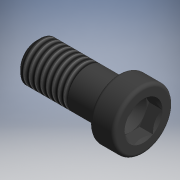
# Autodesk Inventor part: DIN-6912 - M12x25(F)
Saved by Autodesk Inventor 2017.3 (Build 213256000, 256)
## iProperties
Part Number: DIN-6912 - M12x25(F)
Material: Generic
Catalog Web Link: www.cadenas.de
Description: DIN-6912-Hexagon socket head cap screw with centre hole and low head
Vendor: FESTO
Document SubType Name: Modeling
Designer: partserver
Manufacturer: FESTO
Mass: 4.1242 g
Surface Area: 20.1844 cm^2
Volume: 4.1242 cm^3
Density: 1 g/cm^3
Appearance: PSOLRGB-80-80-80
Category: PARTsolutions
Company: FESTO
Title: DIN-6912 - M12x25(F)
Author: Cadenas PARTsolutions
Comments: Hexagon socket head cap screw with centre hole and low head
PSOL_IDENT_0: {$CADENAS_DATA\23d-libs\festo\zyl_zubeh\din_6912\din_6912.prj},183 {VTYP=3D},{NB=DIN-6912 - M12x25(F
PSOL_IDENT_1: )},{LINA=DIN-6912 - M12x25(F)},{NN=DIN-6912},{DATE=16.11.2017 11:29:57},{GEOMDATE=16.11.2017 11:29:4
PSOL_IDENT_2: 4},{VERSION=},{LINEID=550},{WBVAR=},{WBNUMERIC=}  {NB=DIN-6912 - M12x25(F)},{LINA=DIN-6912 - M12x25(
PSOL_IDENT_3: F)},{KT=L},{IDNR=},{NENN=M12x25},{D=12.000},{L=25.000},{DK=9.853},{LS=4.200},{LG=9.500},{DK1=18.000}
PSOL_IDENT_4: ,{DH=6.000},{K=7.500},{R=0.600},{V=1.000},{S=10.000},{T1=4.000},{T2=9.000},{F=1.450},{DA=13.700},{DW=
PSOL_IDENT_5: 17.030}
NB: DIN-6912 - M12x25(F)
NN: DIN-6912
NT: Hexagon socket head cap screw with centre hole and low head
NBSYN: DIN-6912 - $NENN.(F)
LINA: DIN-6912 - M12x25(F)
CATALOG: Festo
ROWDESC: M12x25
D: 12
L: 25
DK: 9.853
LS: 4.2
LG: 9.5
DK1: 18
DH: 6
K: 7.5
R: 0.6
V: 1
S: 10
T1: 4
T2: 9
F: 1.45
DA: 13.7
DW: 17.03
SUPPLIER: FESTO
ARTICLENO: DIN-6912 - M12x25(F)
BOMINFO: DIN-6912 - M12x25(F)
CREATOR: CADENAS GmbH
Autodesk Inventor part; units mm, degrees
sketch "Sketch_1" plane through (0, 0, 0) normal (0, 0, 1) x (1, 0, 0)
  line L0 (25, 0) -> (4.5, 0)
  line L1 (4.5, 0) -> (1.5, 3)
  line L2 (1.5, 3) -> (-1.5, 3)
  line L3 (-1.5, 3) -> (-3.5, 5)
  line L4 (-3.5, 5) -> (-6.7265, 5)
  line L5 (-6.7265, 5) -> (-7.5, 5.7735)
  line L6 (-7.5, 5.7735) -> (-7.5, 8)
  arc A0 (-6.5, 9) -> (-7.5, 8) centre (-6.5, 8) ccw
  line L7 (-6.5, 9) -> (-1, 9)
  arc A1 (0, 8) -> (-1, 9) centre (-1, 8) ccw
  line L8 (0, 8) -> (0, 6)
  line L9 (0, 6) -> (23.9265, 6)
  line L10 (23.9265, 6) -> (25, 4.9265)
  line L11 (25, 4.9265) -> (25, 0)
  line L12 (25, 0) -> (4.5, 0)
  constraints: 26 end point, 4 point on circle, 2 centre point
revolve "Revolution1" add sketch "Sketch_1" angle 360 about axis through (25, 0, 0) along (-1, 0, 0)
thread "Thread1" size "M12x1.75" class "6g" standard "ISO Metric profile" length 14.4265
sketch "Sketch_2" plane through (-7.5, 0, 0) normal (1, 0, 0) x (0, 0, -1)
  line L0 (-5, -2.8868) -> (0, -5.7735)
  line L1 (0, -5.7735) -> (5, -2.8868)
  line L2 (5, -2.8868) -> (5, 2.8868)
  line L3 (5, 2.8868) -> (0, 5.7735)
  line L4 (0, 5.7735) -> (-5, 2.8868)
  line L5 (-5, 2.8868) -> (-5, -2.8868)
  constraints: 12 end point
extrude "Extrusion1" cut sketch "Sketch_2" along normal blind 4
ref_plane "MONTAGE_XY" through (0, 0, 0) normal (1, 0, 0) x (0, 0, -1)
ref_plane "MONTAGE_YZ" through (0, 0, 0) normal (0, 0, -1) x (0, 1, 0)
ref_plane "MONTAGE_ZX" through (0, 0, 0) normal (0, 1, 0) x (1, 0, 0)
ref_plane "Schrauben_punkt_XY" through (25, 0, 0) normal (-1, 0, 0) x (0, 0, -1)
ref_plane "Schrauben_punkt_YZ" through (25, 0, 0) normal (0, 0, -1) x (0, -1, 0)
ref_plane "Schrauben_punkt_ZX" through (25, 0, 0) normal (0, -1, 0) x (-1, 0, 0)
body "Solid1"
